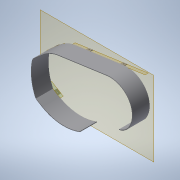
# Autodesk Inventor part: ChainGuard
Saved by Autodesk Inventor 2021 (Build 250183000, 183)
## iProperties
Created: 2020-10-28
Part Number: ChainGuard
Material: Generic
Document SubType Name: Modeling
Designer: PhotonUser
Density: 1 g/cm^3
Appearance: Default
Author: PhotonUser
Autodesk Inventor part; units mm, degrees
ref_plane "YZ Plane" through (0, 0, 0) normal (1, 0, 0) x (0, 1, 0)
ref_plane "XZ Plane" through (0, 0, 0) normal (0, 1, 0) x (-1, 0, 0)
ref_plane "XY Plane" through (0, 0, 0) normal (0, 0, 1) x (1, 0, 0)
ref_plane "Work Plane1" through (0, 0, 0) normal (0, 0, 1) x (1, 0, 0)
sketch "Sketch1" plane through (0, 0, 0) normal (0, 0, 1) x (1, 0, 0)
  line L0 (-148.1629, -85.4758) -> (-100.138, -114.5537)
  arc A0 (-30.3276, 119.385) -> (-94.7251, 90.539) centre (-12.6526, -6.379) ccw
  line L1 (-94.7251, 90.539) -> (-158.4791, 36.5506)
  line L2 (267.4038, 161.2284) -> (-30.3276, 119.385)
  arc A1 (285.61, 2.6867) -> (293.3792, 54.1689) centre (225.4026, 38.1) ccw
  line L3 (293.3792, 54.1689) -> (297.7515, 151.832)
  line L4 (297.7015, -118.5771) -> (285.61, 2.6867)
  line L5 (-144.1535, 48.6818) -> (-94.7251, 90.539)
  line L6 (-130.3534, -96.259) -> (-100.138, -114.5537)
  line L7 (-30.3276, 119.385) -> (187.1449, 149.9488)
  arc A2 (285.61, 2.6867) -> (187.1449, 149.9488) centre (200.8332, 52.5515) ccw
  arc A3 (240.6498, -30.0656) -> (285.61, 2.6867) centre (225.4026, 38.1) ccw
  arc A4 (-30.3276, 119.385) -> (-94.7251, 90.539) centre (-12.6526, -6.379) ccw
  arc A5 (-144.1535, 48.6818) -> (-130.3534, -96.259) centre (70.4605, -4.0117) ccw
  arc A6 (-100.138, -114.5537) -> (65.2631, -125.7611) centre (-5.7133, 52.8688) ccw
  arc A7 (-101.4508, -116.7993) -> (66.2235, -128.1783) centre (-5.7133, 52.8688) ccw
  line L8 (-101.4508, -116.7993) -> (-132.3814, -98.0717)
  arc A8 (-146.4762, 50.1231) -> (-132.3814, -98.0717) centre (70.4605, -4.0117) ccw
  line L9 (-146.4762, 50.1231) -> (-96.406, 92.5238)
  arc A9 (-30.6896, 121.9607) -> (-96.406, 92.5238) centre (-12.6526, -6.379) ccw
  line L10 (-30.6896, 121.9607) -> (186.7829, 152.5244)
  arc A10 (287.8519, 1.3681) -> (186.7829, 152.5244) centre (200.8332, 52.5515) ccw
  arc A11 (241.2176, -32.6038) -> (287.8519, 1.3681) centre (225.4026, 38.1) ccw
  line L11 (65.2631, -125.7611) -> (66.2235, -128.1783)
  line L12 (240.6498, -30.0656) -> (241.2176, -32.6038)
extrude "Extrusion1" add sketch "Sketch1" along normal blind 76.2 contours L0 A6 L11 A7 L8 A8 | L0 A8 L1 A5 | L1 A8 L9 A9 L10 A10 L2 A0 | L2 A10 L3 A2 | L3 A10 A11 L4 A2 | L4 A11 L12 A3
fillet "Fillet1" radius 25.4 2 edges at (-146.4762, 50.1231, 38.1) (-132.3814, -98.0717, 38.1)
ref_plane "Work Plane2" through (-66.6974, 114.2736, 0) normal (-0.1391731, 0.9902681, 0) x (-0.9902681, -0.1391731, 0)
sketch "Sketch2" plane through (-66.6974, 114.2736, 0) normal (-0.1391731, 0.9902681, 0) x (-0.9902681, -0.1391731, 0)
  circle A0 centre (-93.8772, -6.35) radius 2.4892 projected
  circle A1 centre (-249.4522, -6.35) radius 2.4892 projected
  line L0 (-468.6819, 0) -> (219.5709, 0) projected
  line L1 (-36.7272, -12.7) -> (-337.3845, -12.7) projected
  line L2 (-36.7272, 0) -> (-256.3369, 0) projected
  line L3 (-102.8977, 0) -> (-102.8977, -12.7)
  line L4 (-83.8477, -12.7) -> (-102.8977, -12.7)
  line L5 (-83.8477, -12.7) -> (-83.8477, 0)
  circle A2 centre (-93.8772, -6.35) radius 2.4892
  line L6 (-16.5377, -12.7) -> (-16.5377, 0)
  circle A3 centre (-249.4522, -6.35) radius 2.4892
  line L7 (-354.6914, 0) -> (-256.3369, 0) projected
  line L8 (-257.8377, -12.7) -> (-238.7877, -12.7)
  line L9 (-238.7877, -12.7) -> (-238.7877, 0)
  line L10 (-257.8377, -12.7) -> (-257.8377, 0)
  line L11 (-238.7877, 0) -> (-257.8377, 0)
  line L12 (-83.8477, 0) -> (-102.8977, 0)
  line L13 (-97.2698, 0) -> (-97.2698, 76.2) projected
  point P0 (-50.1445, 0)
  point P1 (-333.3488, 0)
  dimension "d7" = 19.05
  dimension "d8" = 67.31
  dimension "d9" = 135.89
  dimension "d10" = 19.05
  constraints: 18 end point, 8 point on line, 4 vertical, 2 centre point, 2 coincident, 2 collinear, 2 concentric, 2 perpendicular, 3 other
  measures "d7" distance between parallel lines of L5 L3
  measures "d8" distance between parallel lines of L5 L6
  measures "d9" distance between parallel lines of L9 L3
  measures "d10" distance from line of L8.start L9
extrude "Extrusion2" add sketch "Sketch2" along normal blind 2.601 contours L0 L9 L1 L10 | L0 L5 L1 L3
ref_plane "Work Plane3" through (-158.4791, 36.5506, 0) normal (-0.6462406, 0.7631337, 0) x (-0.7631337, -0.6462406, 0)
sketch "Sketch3" plane through (-158.4791, 36.5506, 0) normal (-0.6462406, 0.7631337, 0) x (-0.7631337, -0.6462406, 0)
  line L0 (-534.4471, 0) -> (218.8882, 0) projected
  line L1 (0, -12.7) -> (-83.5423, -12.7) projected
  circle A0 centre (-50.8, -6.35) radius 2.4892 projected
  circle A1 centre (-50.8, -6.35) radius 2.4892
  line L2 (-83.5423, 0) -> (-26.3919, 0) projected
  line L3 (-40.767, 0) -> (-40.767, -12.7)
  line L4 (-40.767, -12.7) -> (-60.833, -12.7)
  line L5 (-60.833, -12.7) -> (-60.833, 0)
  line L6 (-60.833, 0) -> (-40.767, 0)
  point P0 (-97.3203, 0)
  point P1 (-60.833, 0)
  point P2 (-40.767, 0)
  dimension "d13" = 10.033
  dimension "d14" = 10.033
  constraints: 8 end point, 4 point on line, 1 centre point, 1 coincident, 1 collinear, 1 concentric, 1 perpendicular, 1 vertical
  measures "d13" distance from line of L3 A0.centre
  measures "d14" distance from line of L5 A0.centre
extrude "Extrusion3" add sketch "Sketch3" along normal blind 2.601
ref_plane "Work Plane4" through (-28.5974, -157.8697, 0) normal (-0.5179348, -0.8554201, 0) x (0.8554201, -0.5179348, 0)
sketch "Sketch4" plane through (-28.5974, -157.8697, 0) normal (-0.5179348, -0.8554201, 0) x (0.8554201, -0.5179348, 0)
  line L0 (-83.6321, -12.7) -> (-139.7741, -12.7) projected
  line L1 (-83.6321, 0) -> (-118.9545, 0) projected
  circle A0 centre (-102.9399, -6.35) radius 2.4892 projected
  circle A1 centre (-102.9399, -6.35) radius 2.4892
  line L2 (-92.9069, -12.7) -> (-92.9069, 0)
  line L3 (-92.9069, 0) -> (-112.9729, 0)
  line L4 (-185.2265, 0) -> (-185.2265, 76.2) projected
  line L5 (-112.9729, 0) -> (-112.9729, -12.7)
  line L6 (-92.9069, -12.7) -> (-112.9729, -12.7)
  point P0 (-57.3034, 0)
  dimension "d19" = 10.033
  dimension "d21" = 10.033
  constraints: 8 end point, 4 point on line, 2 perpendicular, 1 centre point, 1 coincident, 1 collinear, 1 concentric
  measures "d19" distance from line of L2 A0.centre
  measures "d21" horizontal distance of L3.end A0.centre
extrude "Extrusion4" add sketch "Sketch4" along normal blind 2.601
body "Solid1"
